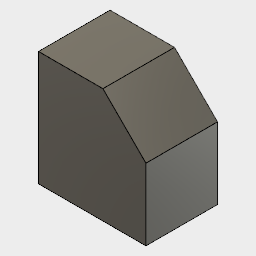
C04-W4-OE-01 (Autodesk Fusion 360 design; units mm, degrees)
Autodesk Fusion 360 part; units mm, degrees
sketch "Sketch1" plane through (0, 0, 0) normal (0, 0, 1) x (1, 0, 0)
  line L0 (0, 0) -> (-75, 0)
  line L1 (-75, 0) -> (-75, 80)
  line L2 (-75, 80) -> (-30, 80)
  line L3 (-30, 80) -> (0, 50)
  line L4 (0, 50) -> (0, 0)
  dimension "d1" = 75
  dimension "d2" = 80
  dimension "d3" = 135
  dimension "d4" = 50
  measures "d1" distance of L0.start L0.end
  measures "d2" distance of L0.end L1.end
  measures "d3" angle of L2 L3
  measures "d4" distance of L0.start L3.end
extrude "Extrude1" add sketch "Sketch1" along normal mid plane 50
